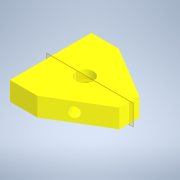
# Autodesk Inventor part: 30_Cube_Z_Focus_Drylin_NEMA_slide_part1
Saved by Autodesk Inventor 2022 (Build 260153000, 153)
## iProperties
Created: 2021-05-05
Part Number: 30_Cube_Z_Focus_Drylin_NEMA_slide_part1
Material: Generic
Document SubType Name: Modeling
Designer: diederichbenedict
Density: 1 g/cm^3
Appearance: Smooth - Yellow
Author: diederichbenedict
Autodesk Inventor part; units mm, degrees
ref_plane "YZ Plane" through (0, 0, 0) normal (1, 0, 0) x (0, 1, 0)
ref_plane "XZ Plane" through (0, 0, 0) normal (0, 1, 0) x (-1, 0, 0)
ref_plane "XY Plane" through (0, 0, 0) normal (0, 0, 1) x (1, 0, 0)
sketch "Sketch1" plane through (0, 0, 0) normal (0, 1, 0) x (-1, 0, 0)
  line L0 (-13, -11.9282) -> (10, -11.9282)
  line L1 (10, -11.9282) -> (10, 11.9282)
  line L2 (10, 11.9282) -> (-13, 11.9282)
  line L3 (-13, 11.9282) -> (-13, -11.9282)
  circle A0 centre (-8, 0) radius 4
  circle A1 centre (4, -6.9282) radius 4
  circle A2 centre (4, 6.9282) radius 4
  circle A3 centre (0, 0) radius 8 construction
  circle A4 centre (0, 0) radius 1.75
  dimension "d11" = 16
  dimension "d2" = 8
  dimension "d6" = 360
  dimension "d8" = 6
  dimension "d9" = 5
  dimension "d12" = 5
  dimension "d13" = 5
  dimension "d35" = 3.5
  constraints: 8 end point, 4 centre point, 3 coincident, 2 parallel, 1 horizontal, 1 horizontal alignment, 1 perpendicular, 9 other
  measures "d2" diameter of A0
  measures "d8" distance from line of A2.centre L1
  measures "d9" distance from line of L3 A0.centre
  measures "d12" distance from line of L2 A2.centre
  measures "d13" distance from line of L0 A1.centre
  measures "d35" diameter of A4
extrude "Extrusion1" add sketch "Sketch1" along normal blind 3
sketch "Sketch2" plane through (0, 3, 0) normal (0, 1, 0) x (1, 0, 0)
  circle A0 centre (-4, -6.9282) radius 4 projected
  circle A1 centre (-4, 6.9282) radius 4 projected
  circle A2 centre (8, 0) radius 4 projected
  line L0 (13, 11.9282) -> (-10, 11.9282) projected
  line L1 (-10, 11.9282) -> (-10, -11.9282) projected
  line L2 (-10, -11.9282) -> (13, -11.9282) projected
  line L3 (13, -11.9282) -> (13, 11.9282) projected
  circle A3 centre (0, 0) radius 2.5
  dimension "d16" = 5
  constraints: 1 centre point, 1 coincident
  measures "d16" diameter of A3
extrude "Extrusion2" add sketch "Sketch2" along normal blind 2.5 contours A0 | A1 | A2 | L3 L2 L1 L0
sketch "Sketch3" plane through (0, 0, 0) normal (0, -1, 0) x (1, 0, 0)
  circle A0 centre (-4, 6.9282) radius 4 projected
  circle A1 centre (-4, -6.9282) radius 4 projected
  circle A2 centre (8, 0) radius 4 projected
  line L0 (13, -11.9282) -> (-10, -11.9282) projected
  line L1 (13, 11.9282) -> (13, -11.9282) projected
  line L2 (-10, 11.9282) -> (13, 11.9282) projected
  line L3 (-10, -11.9282) -> (-10, 11.9282) construction
  line L4 (-2, 11.9282) -> (13, 2.9282)
  line L5 (13, 11.9282) -> (13, -11.9282) projected
  line L6 (13, -2.9282) -> (-2, -11.9282)
  point P0 (0, 0)
  dimension "d19" = 9
  dimension "d20" = 9
  dimension "d21" = 15
  dimension "d22" = 15
  constraints: 4 end point, 4 point on line
  measures "d19" distance from line of L2 L4.end
  measures "d20" distance from line of L0 L6.start
  measures "d21" distance from line of L6.end L1
  measures "d22" distance from line of L1 L4.start
extrude "Extrusion3" cut sketch "Sketch3" against normal through all contours L4 L2 L1 | L0 L6 L1
sketch "Skizze10" plane through (-2, 0, 11.9282) normal (0.5145, 0, 0.8575) x (0.8575, 0, -0.5145)
  line L0 (9.602, 0) -> (6.102, 0) projected
  line L1 (9.602, 0) -> (9.602, 3) projected
  line L2 (6.102, 0) -> (6.102, 3) projected
  circle A0 centre (7.852, 2.6816) radius 1.45
  point P0 (7.852, 0)
  dimension "d42" = 2.9
  constraints: 1 centre point
  measures "d42" diameter of A0
extrude "Extrusion9" cut sketch "Skizze10" against normal up to surface
ref_plane "Arbeitsebene1" through (-10, 0, 0) normal (0, 0, 1) x (1, 0, 0)
mirror "Spiegeln1" about plane through (-10, 0, 0) normal (0, 0, 1) of "Extrusion9"
equation "\"d12\" = d9"
equation "\"d13\" = d9"
equation "\"d43\" = d42"
body "Solid1"
